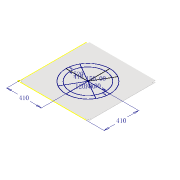
# Autodesk Inventor part: 底板
Saved by Autodesk Inventor 2021 (Build 250183000, 183)
## iProperties
Created: 2025-04-16
Part Number: 底板
Material: 常规
Document SubType Name: Modeling
Designer: 86155
Density: 1 g/cm^3
Appearance: 默认
Author: 86155
Autodesk Inventor part; units mm, degrees
ref_plane "YZ Plane" through (0, 0, 0) normal (1, 0, 0) x (0, 1, 0)
ref_plane "XZ Plane" through (0, 0, 0) normal (0, 1, 0) x (-1, 0, 0)
ref_plane "XY Plane" through (0, 0, 0) normal (0, 0, 1) x (1, 0, 0)
sketch "草图1" plane through (0, 0, 0) normal (0, 1, 0) x (-1, 0, 0)
  line L0 (0, 0) -> (-820, 0)
  line L1 (-820, 0) -> (-820, -820)
  line L2 (-820, -820) -> (0, -820)
  line L3 (0, -820) -> (0, 0)
  dimension "d0" = 820
  dimension "d1" = 820
  constraints: 8 end point, 2 parallel, 1 horizontal, 1 perpendicular
  measures "d0" distance of L2.end L1.end
  measures "d1" distance of L1.end L0.end
extrude "拉伸1" add sketch "草图1" along normal blind 5
sketch "草图2" plane through (0, 5, 0) normal (0, 1, 0) x (1, 0, 0)
  line L0 (0, 0) -> (820, 0) projected
  line L1 (0, 0) -> (20, 0)
  line L2 (20, 0) -> (20, 20)
  line L3 (20, 20) -> (0, 20)
  line L4 (0, 20) -> (0, 0)
  line L5 (820, 0) -> (800, 0)
  line L6 (800, 0) -> (800, 20)
  line L7 (800, 20) -> (820, 20)
  line L8 (820, 20) -> (820, 0)
  line L9 (820, 820) -> (0, 820) projected
  line L10 (820, 820) -> (800, 820)
  line L11 (800, 820) -> (800, 800)
  line L12 (800, 800) -> (820, 800)
  line L13 (820, 800) -> (820, 820)
  line L14 (0, 820) -> (20, 820)
  line L15 (20, 820) -> (20, 800)
  line L16 (20, 800) -> (0, 800)
  line L17 (0, 800) -> (0, 820)
  dimension "d4" = 20
  dimension "d5" = 20
  dimension "d6" = 20
  dimension "d7" = 20
  dimension "d8" = 20
  dimension "d9" = 20
  dimension "d10" = 20
  dimension "d11" = 20
  constraints: 32 end point, 8 parallel, 4 horizontal, 4 perpendicular
  measures "d4" distance of L3.end L2.end
  measures "d5" distance of L2.end L1.end
  measures "d6" distance of L6.end L7.end
  measures "d7" distance of L5.end L6.end
  measures "d8" distance of L12.end L11.end
  measures "d9" distance of L11.end L10.end
  measures "d10" distance of L15.end L16.end
  measures "d11" distance of L14.end L15.end
extrude "拉伸2" cut sketch "草图2" against normal blind 5
sketch "草图3" plane through (0, 5, 0) normal (0, 1, 0) x (1, 0, 0)
  line L0 (20, 0) -> (800, 0) projected
  line L1 (0, 800) -> (0, 20) projected
  line L2 (820, 20) -> (820, 800) projected
  line L3 (800, 820) -> (20, 820) projected
  point P0 (0, 0)
  point P1 (40, 10)
  point P2 (780, 10)
  point P3 (810, 780)
  point P4 (780, 810)
  point P5 (40, 810)
  point P6 (10, 780)
  point P7 (10, 40)
  point P8 (810, 40)
  dimension "d14" = 10
  dimension "d15" = 40
  dimension "d16" = 10
  dimension "d17" = 40
  dimension "d18" = 10
  dimension "d19" = 40
  dimension "d20" = 10
  dimension "d21" = 40
  dimension "d22" = 10
  dimension "d23" = 40
  dimension "d24" = 10
  dimension "d25" = 40
  dimension "d26" = 10
  dimension "d27" = 40
  dimension "d28" = 10
  dimension "d29" = 40
  measures "d14" distance from line of L0 point (40, 10)
  measures "d15" distance from line of L1 point (40, 10)
  measures "d16" distance from line of L0 point (780, 10)
  measures "d17" distance from line of L2 point (780, 10)
  measures "d18" distance from line of L2 point (810, 40)
  measures "d19" distance from line of L0 point (810, 40)
  measures "d20" distance from line of L2 point (810, 780)
  measures "d21" distance from line of L3 point (810, 780)
  measures "d22" distance from line of L3 point (780, 810)
  measures "d23" distance from line of L2 point (780, 810)
  measures "d24" distance from line of L3 point (40, 810)
  measures "d25" distance from line of L1 point (40, 810)
  measures "d26" distance from line of L1 point (10, 780)
  measures "d27" distance from line of L3 point (10, 780)
  measures "d28" distance from line of L1 point (10, 40)
  measures "d29" distance from line of L0 point (10, 40)
hole "孔1" at (40, 5, -10) at (780, 5, -10) at (810, 5, -780) at (780, 5, -810) at (40, 5, -810) at (10, 5, -780) at (10, 5, -40) at (810, 5, -40) direction (0, -1, 0) diameter 4.9587 depth 13.8 tip angle 118 thread size "M5.5x0.5" class "6H" standard "GB Metric profile"
sketch "草图4" plane through (0, 5, 0) normal (0, 1, 0) x (1, 0, 0)
  circle A0 centre (410, 410) radius 260
  circle A1 centre (410, 410) radius 208
  line L0 (0, 800) -> (0, 20) projected
  line L1 (20, 0) -> (800, 0) projected
  line L2 (410, 410) -> (410, 150)
  line L3 (410, 410) -> (280, 184.8334)
  line L4 (410, 410) -> (670, 410) construction
  line L5 (410, 410) -> (410, 670)
  line L6 (410, 410) -> (150, 410)
  line L7 (410, 410) -> (670, 410)
  line L8 (410, 410) -> (540, 635.1666)
  line L9 (410, 410) -> (635.1666, 280)
  line L10 (410, 410) -> (670, 410) construction
  line L11 (410, 410) -> (184.8334, 540)
  line L12 (410, 410) -> (670, 410) construction
  circle A2 centre (410, 410) radius 240
  line L13 (410, 410) -> (178.1778, 472.1166)
  line L14 (410, 410) -> (650, 410) construction
  point P0 (0, 0)
  point P1 (347.8834, 178.1778)
  point P2 (347.8834, 178.1778)
  point P3 (641.8222, 347.8834)
  point P4 (641.8222, 347.8834)
  point P5 (472.1166, 641.8222)
  point P6 (472.1166, 641.8222)
  dimension "d37" = 520
  dimension "d44" = 480
  dimension "d38" = 416
  dimension "d39" = 410
  dimension "d40" = 410
  dimension "d41" = 120
  dimension "d42" = 30
  dimension "d43" = 150
  dimension "d45" = 165
  dimension "d48" = 360
  constraints: 26 end point, 6 coincident, 4 equal length, 4 horizontal, 1 centre point, 1 collinear, 1 perpendicular, 1 vertical, 21 other
  measures "d38" diameter of A1
  measures "d39" distance from line of L0 point (410, 410)
  measures "d40" distance from line of L1 point (410, 410)
  measures "d41" angle of L3 L4
  measures "d42" angle of L9 L10
  measures "d43" angle of L12 L11
  measures "d45" angle of L14 L13
hole "孔2" at (178.1778, 5, -472.1166) at (347.8834, 5, -178.1778) at (641.8222, 5, -347.8834) at (472.1166, 5, -641.8222) direction (0, -1, 0) diameter 6.647 depth 22.2 tip angle 118 thread size "M8x1.25" designation "M8" class "6H" standard "GB Metric profile"
